y_guide_holder (Autodesk Fusion 360 design; units mm, degrees)
Autodesk Fusion 360 part; units mm, degrees
sketch "Sketch1" plane through (0, 0, 0) normal (0, 1, 0) x (1, 0, 0)
  line L0 (-7.5, 0) -> (-20, 0)
  line L1 (-20, 0) -> (-20, 8)
  line L2 (-20, 8) -> (20, 8)
  line L3 (20, 8) -> (20, 0)
  line L4 (20, 0) -> (7.5, 0)
  arc A0 (-7.5, 0) -> (7.5, 0) centre (0, 0) ccw
  circle A1 centre (0, 0) radius 4
  dimension "d1" = 15
  dimension "d2" = 20
  dimension "d3" = 20
  dimension "d4" = 8
  dimension "d5" = 8
  constraint coincident A0.centre A1.centre
  constraint horizontal L0
  constraint perpendicular L0 L1
  constraint perpendicular L1 L2
  constraint perpendicular L0 L3
  constraint perpendicular L3 L4
  constraint horizontal A0.centre L4.end
  constraint horizontal A0.centre L0.start
  constraint concentric A0 A1
  measures "d1" diameter of A0
  measures "d2" distance of A0.centre L1
  measures "d3" distance of A0.centre L3
  measures "d4" distance of L0.end L1.end
  measures "d5" diameter of A1
extrude "Extrude1" add sketch "Sketch1" along normal blind 30 contours L0 L1 L2 L3 L4 A0 | A1
extrude "Extrude2" cut sketch "Sketch1" along normal blind 15 contours A1
fillet "Fillet1" radius 3 4 edges at (-7.5, 15, 0) (7.5, 15, 0) (20, 15, 0) (-20, 15, 0)
sketch "Sketch2" plane through (0, 0, 0) normal (0, 0, 1) x (-1, 0, 0)
  line L0 (-17, 0) -> (-17, -30)
  line L1 (-17, -30) -> (-10.0623, -30)
  line L2 (-10.0623, -30) -> (-10.0623, 0)
  line L3 (-10.0623, 0) -> (-17, 0)
  circle A0 centre (14, -15) radius 1.6
  circle A1 centre (-14, -15) radius 1.6
  line L4 (10.0623, 0) -> (17, 0)
  dimension "d12" = 3.2
  dimension "d13" = 15
  dimension "d14" = 14
  dimension "d15" = 14
  constraint equal A0 A1
  constraint horizontal A0.centre A1.centre
  measures "d12" diameter of A0
  measures "d13" distance of A0.centre L4
  measures "d14" horizontal distance of origin A0.centre
  measures "d15" horizontal distance of origin A1.centre
extrude "Extrude3" cut sketch "Sketch2" against normal through all contours A0 | A1
fillet "Fillet2" radius 3 9 edges at (-20, 30, -5.5) (-19.1213, 30, -0.8787) (-13.5312, 30, 0) (-8.2695, 30, 0.5946) (0, 30, 7.5) (8.2695, 30, 0.5946) (13.5312, 30, 0) (19.1213, 30, -0.8787) (20, 30, -5.5)
equation "d3 = d2"
equation "d15 = d14"
